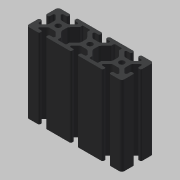
# Autodesk Inventor part: 40-4012-BLACK-FB
Saved by Autodesk Inventor 2013 SP2 (Build 170200200, 200)
## iProperties
Company: 80/20 Inc.
Created: 2014-04-23
Part Number: 40-4012-BLACK-FB
Material: Generic
Document SubType Name: Modeling
Designer: Ross Bowman
Density: 1 g/cm^3
Engineer: Ross Bowman
Catalog Web Link: 8020.net
Vendor: 80/20 Inc.
Mass: 225.385 g
Surface Area: 916.102 cm^2
Volume: 225.385 cm^3
Material: 6105-T5 Aluminum
Author: Ross Bowman
Keywords: 80/20 , 8020 , T-Slot , Extrusion
Autodesk Inventor part; units mm, degrees
ref_plane "YZ Plane" through (0, 0, 0) normal (1, 0, 0) x (0, 1, 0)
ref_plane "XZ Plane" through (0, 0, 0) normal (0, 1, 0) x (-1, 0, 0)
ref_plane "XY Plane" through (0, 0, 0) normal (0, 0, 1) x (1, 0, 0)
sketch "Sketch1" plane through (0, 0, 0) normal (0, 0, 1) x (1, 0, 0)
  circle A0 centre (40, 0) radius 3.4
  line L0 (9.0912, -6.0165) -> (14.2186, -11.1439)
  arc A1 (7.7, -2.6578) -> (9.0912, -6.0165) centre (12.45, -2.6578) ccw
  line L1 (7.7, 2.6265) -> (7.7, -2.6578)
  arc A2 (9.4012, 5.7139) -> (7.7, 2.6265) centre (12.4138, 2.0415) ccw
  line L2 (14.6946, 11.0074) -> (9.4012, 5.7139)
  arc A3 (14.6946, 11.0074) -> (15.0666, 11.9054) centre (13.7966, 11.9054) ccw
  line L3 (15.0666, 14.2735) -> (15.0666, 11.9054)
  arc A4 (16.3366, 15.68) -> (15.0666, 14.2735) centre (16.3292, 14.41) ccw
  line L4 (23.6634, 15.68) -> (16.3366, 15.68)
  arc A5 (24.9334, 14.41) -> (23.6634, 15.68) centre (23.6634, 14.41) ccw
  line L5 (24.9334, 12.0419) -> (24.9334, 14.41)
  arc A6 (24.9334, 12.0419) -> (25.3054, 11.1439) centre (26.2034, 12.0419) ccw
  line L6 (30.5988, 5.8505) -> (25.3054, 11.1439)
  arc A7 (32.3, 2.6265) -> (30.5988, 5.8505) centre (27.57, 2.1914) ccw
  line L7 (32.3, -2.6578) -> (32.3, 2.6265)
  arc A8 (30.9088, -6.0165) -> (32.3, -2.6578) centre (27.55, -2.6578) ccw
  line L8 (25.7814, -11.1439) -> (30.9088, -6.0165)
  arc A9 (25.7814, -11.1439) -> (25.4094, -12.0419) centre (26.6794, -12.0419) ccw
  line L9 (25.4094, -14.41) -> (25.4094, -12.0419)
  arc A10 (24.1394, -15.68) -> (25.4094, -14.41) centre (24.1394, -14.41) ccw
  line L10 (15.8606, -15.68) -> (24.1394, -15.68)
  arc A11 (14.5906, -14.41) -> (15.8606, -15.68) centre (15.8606, -14.41) ccw
  line L11 (14.5906, -12.0419) -> (14.5906, -14.41)
  arc A12 (14.5906, -12.0419) -> (14.2186, -11.1439) centre (13.3206, -12.0419) ccw
  circle A13 centre (0, 0) radius 3.4
  line L12 (-30.9088, -5.384) -> (-25.7814, -10.5113)
  arc A14 (-32.3, -2.0252) -> (-30.9088, -5.384) centre (-27.55, -2.0252) ccw
  line L13 (-32.3, 3.2591) -> (-32.3, -2.0252)
  arc A15 (-30.5988, 6.3465) -> (-32.3, 3.2591) centre (-27.5862, 2.6741) ccw
  line L14 (-25.3054, 11.6399) -> (-30.5988, 6.3465)
  arc A16 (-25.3054, 11.6399) -> (-24.9334, 12.538) centre (-26.2034, 12.538) ccw
  line L15 (-24.9334, 14.9061) -> (-24.9334, 12.538)
  arc A17 (-23.6634, 15.68) -> (-24.9334, 14.9061) centre (-23.7626, 14.4139) ccw
  line L16 (-16.3366, 15.68) -> (-23.6634, 15.68)
  arc A18 (-15.0666, 14.41) -> (-16.3366, 15.68) centre (-16.3366, 14.41) ccw
  line L17 (-15.0666, 12.0419) -> (-15.0666, 14.41)
  arc A19 (-15.0666, 12.0419) -> (-14.6946, 11.1439) centre (-13.7966, 12.0419) ccw
  line L18 (-9.4012, 5.8505) -> (-14.6946, 11.1439)
  arc A20 (-7.7, 2.6265) -> (-9.4012, 5.8505) centre (-12.43, 2.1914) ccw
  line L19 (-7.7, -2.6578) -> (-7.7, 2.6265)
  arc A21 (-9.0912, -6.0165) -> (-7.7, -2.6578) centre (-12.45, -2.6578) ccw
  line L20 (-14.2186, -11.1439) -> (-9.0912, -6.0165)
  arc A22 (-14.2186, -11.1439) -> (-14.5906, -12.0419) centre (-13.3206, -12.0419) ccw
  line L21 (-14.5906, -14.41) -> (-14.5906, -12.0419)
  arc A23 (-15.8606, -15.68) -> (-14.5906, -14.41) centre (-15.8606, -14.41) ccw
  line L22 (-24.1394, -15.68) -> (-15.8606, -15.68)
  arc A24 (-25.4094, -14.41) -> (-24.1394, -15.68) centre (-24.1394, -14.41) ccw
  line L23 (-25.4094, -11.4093) -> (-25.4094, -14.41)
  arc A25 (-25.4094, -11.4093) -> (-25.7814, -10.5113) centre (-26.6794, -11.4093) ccw
  circle A26 centre (-40, 0) radius 3.4
  arc A27 (-5.63, -20) -> (-4.06, -18.43) centre (-5.63, -18.43) ccw
  line L24 (-4.06, -18.43) -> (-4.06, -17.2093)
  arc A28 (-4.06, -17.2093) -> (-5.63, -15.68) centre (-5.6295, -17.25) ccw
  line L25 (-5.63, -15.68) -> (-8.7404, -15.68)
  arc A29 (-10.3104, -14.11) -> (-8.7404, -15.68) centre (-8.7404, -14.11) ccw
  line L26 (-10.3104, -14.11) -> (-10.3104, -13.7197)
  arc A30 (-10.0878, -13.1823) -> (-10.3104, -13.7197) centre (-9.5504, -13.7197) ccw
  line L27 (-10.0878, -13.1823) -> (-6.3105, -9.405)
  arc A31 (-3.3425, -7.7407) -> (-6.3105, -9.405) centre (-2.6575, -12.4411) ccw
  line L28 (-3.3425, -7.7407) -> (3.3406, -7.7407)
  arc A32 (6.3086, -9.405) -> (3.3406, -7.7407) centre (2.6556, -12.4411) ccw
  line L29 (6.3086, -9.405) -> (10.037, -13.1334)
  arc A33 (10.2596, -13.6708) -> (10.037, -13.1334) centre (9.4996, -13.6708) ccw
  line L30 (10.2596, -13.6708) -> (10.2596, -14.11)
  arc A34 (8.6896, -15.68) -> (10.2596, -14.11) centre (8.6896, -14.11) ccw
  line L31 (8.6896, -15.68) -> (5.5792, -15.68)
  arc A35 (5.5792, -15.68) -> (4.0092, -17.2093) centre (5.5787, -17.25) ccw
  line L32 (4.0092, -17.2093) -> (4.0092, -18.43)
  arc A36 (4.0092, -18.43) -> (5.5792, -20) centre (5.5792, -18.43) ccw
  line L33 (5.5792, -20) -> (34.3192, -20)
  arc A37 (34.3192, -20) -> (35.8892, -18.43) centre (34.3192, -18.43) ccw
  line L34 (35.8892, -18.43) -> (35.8892, -17.2093)
  arc A38 (35.8892, -17.2093) -> (34.3192, -15.68) centre (34.3197, -17.25) ccw
  line L35 (34.3192, -15.68) -> (31.2088, -15.68)
  arc A39 (29.6886, -14.0552) -> (31.2088, -15.68) centre (31.2577, -14.1108) ccw
  line L36 (29.6886, -14.0552) -> (29.6886, -13.6708)
  arc A40 (29.9112, -13.1334) -> (29.6886, -13.6708) centre (30.4486, -13.6708) ccw
  line L37 (29.9112, -13.1334) -> (33.6397, -9.405)
  arc A41 (36.6076, -7.7407) -> (33.6397, -9.405) centre (37.2927, -12.4411) ccw
  line L38 (36.6076, -7.7407) -> (43.2907, -7.7407)
  arc A42 (46.2587, -9.405) -> (43.2907, -7.7407) centre (42.6057, -12.4411) ccw
  line L39 (46.2587, -9.405) -> (50.036, -13.1823)
  arc A43 (50.2586, -13.7197) -> (50.036, -13.1823) centre (49.4986, -13.7197) ccw
  line L40 (50.2586, -13.7197) -> (50.2586, -14.0552)
  arc A44 (48.6896, -15.68) -> (50.2586, -14.0552) centre (48.6896, -14.11) ccw
  line L41 (48.6896, -15.68) -> (45.5792, -15.68)
  arc A45 (45.5792, -15.68) -> (44.0092, -17.2093) centre (45.5787, -17.25) ccw
  line L42 (44.0092, -17.2093) -> (44.0092, -18.4389)
  arc A46 (44.0092, -18.4389) -> (45.7462, -20) centre (45.5792, -18.4389) ccw
  line L43 (45.7462, -20) -> (57.0066, -20)
  arc A47 (57.0066, -20) -> (60, -16.83) centre (56.83, -16.8349) ccw
  line L44 (60, -16.83) -> (60, -5.5696)
  arc A48 (60, -5.5696) -> (58.43, -3.9996) centre (58.43, -5.5696) ccw
  line L45 (58.43, -3.9996) -> (57.25, -3.9996)
  arc A49 (57.25, -3.9996) -> (55.68, -5.5696) centre (57.25, -5.5696) ccw
  line L46 (55.68, -5.5696) -> (55.68, -8.4722)
  arc A50 (54.111, -10.097) -> (55.68, -8.4722) centre (54.111, -8.527) ccw
  line L47 (54.111, -10.097) -> (53.4665, -10.097)
  arc A51 (52.9291, -9.8744) -> (53.4665, -10.097) centre (53.4665, -9.337) ccw
  line L48 (52.9291, -9.8744) -> (48.9155, -5.8608)
  arc A52 (47.7, -2.502) -> (48.9155, -5.8608) centre (52.4465, -2.6836) ccw
  line L49 (47.7, -2.502) -> (47.7, 2.571)
  arc A53 (49.0111, 5.9564) -> (47.7, 2.571) centre (52.4488, 2.6785) ccw
  line L50 (49.0111, 5.9564) -> (53.1886, 10.1339)
  arc A54 (53.726, 10.3565) -> (53.1886, 10.1339) centre (53.726, 9.5965) ccw
  line L51 (53.726, 10.3565) -> (54.11, 10.3565)
  arc A55 (55.68, 8.7865) -> (54.11, 10.3565) centre (54.11, 8.7865) ccw
  line L52 (55.68, 8.7865) -> (55.68, 5.8839)
  arc A56 (55.68, 5.8839) -> (57.1443, 4.1259) centre (57.2384, 5.693) ccw
  line L53 (57.1443, 4.1259) -> (58.3243, 4.1259)
  arc A57 (58.3243, 4.1259) -> (60, 5.5825) centre (58.4338, 5.692) ccw
  line L54 (60, 5.5825) -> (60, 16.8406)
  arc A58 (60, 16.8406) -> (56.83, 20) centre (56.83, 16.83) ccw
  line L55 (56.83, 20) -> (45.5696, 20)
  arc A59 (45.5696, 20) -> (43.9996, 18.43) centre (45.5696, 18.43) ccw
  line L56 (43.9996, 18.43) -> (43.9996, 17.25)
  arc A60 (43.9996, 17.25) -> (45.5696, 15.68) centre (45.5696, 17.25) ccw
  line L57 (45.5696, 15.68) -> (48.715, 15.68)
  arc A61 (50.285, 14.11) -> (48.715, 15.68) centre (48.715, 14.11) ccw
  line L58 (50.285, 14.11) -> (50.285, 13.6545)
  arc A62 (50.0624, 13.1171) -> (50.285, 13.6545) centre (49.525, 13.6545) ccw
  line L59 (50.0624, 13.1171) -> (45.9081, 8.9628)
  arc A63 (42.5494, 7.7) -> (45.9081, 8.9628) centre (42.6809, 12.4482) ccw
  line L60 (42.5494, 7.7) -> (37.4506, 7.7)
  arc A64 (34.0919, 8.9628) -> (37.4506, 7.7) centre (37.3191, 12.4482) ccw
  line L61 (34.0919, 8.9628) -> (29.9376, 13.1171)
  arc A65 (29.715, 13.6545) -> (29.9376, 13.1171) centre (30.475, 13.6545) ccw
  line L62 (29.715, 13.6545) -> (29.715, 14.11)
  arc A66 (31.285, 15.68) -> (29.715, 14.11) centre (31.285, 14.11) ccw
  line L63 (31.285, 15.68) -> (34.5165, 15.68)
  arc A67 (34.5165, 15.68) -> (36.0865, 17.25) centre (34.5165, 17.25) ccw
  line L64 (36.0865, 17.25) -> (36.0865, 18.43)
  arc A68 (36.0865, 18.43) -> (34.5165, 20) centre (34.5165, 18.43) ccw
  line L65 (34.5165, 20) -> (5.4816, 20)
  arc A69 (5.4816, 20) -> (3.9116, 18.43) centre (5.4816, 18.43) ccw
  line L66 (3.9116, 18.43) -> (3.9116, 17.25)
  arc A70 (3.9116, 17.25) -> (5.4816, 15.68) centre (5.4816, 17.25) ccw
  line L67 (5.4816, 15.68) -> (8.715, 15.68)
  arc A71 (10.285, 14.11) -> (8.715, 15.68) centre (8.715, 14.11) ccw
  line L68 (10.285, 14.11) -> (10.285, 13.6545)
  arc A72 (10.0624, 13.1171) -> (10.285, 13.6545) centre (9.525, 13.6545) ccw
  line L69 (10.0624, 13.1171) -> (5.9081, 8.9628)
  arc A73 (2.5494, 7.7) -> (5.9081, 8.9628) centre (2.6809, 12.4482) ccw
  line L70 (2.5494, 7.7) -> (-2.5494, 7.7)
  arc A74 (-5.9081, 8.9628) -> (-2.5494, 7.7) centre (-2.6809, 12.4482) ccw
  line L71 (-5.9081, 8.9628) -> (-10.0624, 13.1171)
  arc A75 (-10.285, 13.6545) -> (-10.0624, 13.1171) centre (-9.525, 13.6545) ccw
  line L72 (-10.285, 13.6545) -> (-10.285, 14.11)
  arc A76 (-8.715, 15.68) -> (-10.285, 14.11) centre (-8.715, 14.11) ccw
  line L73 (-8.715, 15.68) -> (-5.4835, 15.68)
  arc A77 (-5.4835, 15.68) -> (-3.9135, 17.25) centre (-5.4835, 17.25) ccw
  line L74 (-3.9135, 17.25) -> (-3.9135, 18.43)
  arc A78 (-3.9135, 18.43) -> (-5.4835, 20) centre (-5.4835, 18.43) ccw
  line L75 (-5.4835, 20) -> (-34.5165, 20)
  line L76 (-36.0865, 18.43) -> (-36.0865, 17.2476)
  arc A79 (-36.0865, 17.2476) -> (-34.5165, 15.68) centre (-34.5165, 17.25) ccw
  line L77 (-34.5165, 15.68) -> (-31.285, 15.68)
  arc A80 (-29.715, 14.11) -> (-31.285, 15.68) centre (-31.285, 14.11) ccw
  line L78 (-29.715, 14.11) -> (-29.715, 13.6545)
  arc A81 (-29.9376, 13.1171) -> (-29.715, 13.6545) centre (-30.475, 13.6545) ccw
  line L79 (-29.9376, 13.1171) -> (-34.0919, 8.9628)
  arc A82 (-37.4506, 7.7) -> (-34.0919, 8.9628) centre (-37.3191, 12.4482) ccw
  line L80 (-37.4506, 7.7) -> (-42.5494, 7.7)
  arc A83 (-45.9081, 8.9628) -> (-42.5494, 7.7) centre (-42.6809, 12.4482) ccw
  line L81 (-45.9081, 8.9628) -> (-50.0624, 13.1171)
  arc A84 (-50.285, 13.6545) -> (-50.0624, 13.1171) centre (-49.525, 13.6545) ccw
  line L82 (-50.285, 13.6545) -> (-50.285, 14.11)
  arc A85 (-48.715, 15.68) -> (-50.285, 14.11) centre (-48.715, 14.11) ccw
  line L83 (-48.715, 15.68) -> (-45.5696, 15.68)
  arc A86 (-45.5696, 15.68) -> (-43.9996, 17.25) centre (-45.5696, 17.25) ccw
  line L84 (-43.9996, 17.25) -> (-43.9996, 18.43)
  arc A87 (-43.9996, 18.43) -> (-45.5696, 20) centre (-45.5696, 18.43) ccw
  line L85 (-45.5696, 20) -> (-56.83, 20)
  arc A88 (-56.83, 20) -> (-60, 16.8406) centre (-56.83, 16.83) ccw
  line L86 (-60, 16.8406) -> (-60, 5.5825)
  arc A89 (-60, 5.5825) -> (-58.3243, 4.1259) centre (-58.4338, 5.692) ccw
  line L87 (-58.3243, 4.1259) -> (-57.1443, 4.1259)
  arc A90 (-57.1443, 4.1259) -> (-55.68, 5.8839) centre (-57.2384, 5.693) ccw
  line L88 (-55.68, 5.8839) -> (-55.68, 8.7865)
  arc A91 (-54.11, 10.3565) -> (-55.68, 8.7865) centre (-54.11, 8.7865) ccw
  line L89 (-54.11, 10.3565) -> (-53.726, 10.3565)
  arc A92 (-53.1886, 10.1339) -> (-53.726, 10.3565) centre (-53.726, 9.5965) ccw
  line L90 (-53.1886, 10.1339) -> (-49.0111, 5.9564)
  arc A93 (-47.7, 2.571) -> (-49.0111, 5.9564) centre (-52.4488, 2.6785) ccw
  line L91 (-47.7, 2.571) -> (-47.7, -2.502)
  arc A94 (-48.9155, -5.8608) -> (-47.7, -2.502) centre (-52.4465, -2.6836) ccw
  line L92 (-48.9155, -5.8608) -> (-52.9291, -9.8744)
  arc A95 (-53.4665, -10.097) -> (-52.9291, -9.8744) centre (-53.4665, -9.337) ccw
  line L93 (-53.4665, -10.097) -> (-54.111, -10.097)
  arc A96 (-55.68, -8.4722) -> (-54.111, -10.097) centre (-54.111, -8.527) ccw
  line L94 (-55.68, -8.4722) -> (-55.68, -5.5696)
  arc A97 (-55.68, -5.5696) -> (-57.25, -3.9996) centre (-57.25, -5.5696) ccw
  line L95 (-57.25, -3.9996) -> (-58.43, -3.9996)
  arc A98 (-58.43, -3.9996) -> (-60, -5.5696) centre (-58.43, -5.5696) ccw
  line L96 (-60, -5.5696) -> (-60, -16.83)
  arc A99 (-60, -16.83) -> (-57.0574, -20) centre (-56.83, -16.8382) ccw
  line L97 (-57.0574, -20) -> (-45.797, -20)
  arc A100 (-45.797, -20) -> (-44.06, -18.4389) centre (-45.63, -18.4389) ccw
  line L98 (-44.06, -18.4389) -> (-44.06, -17.25)
  arc A101 (-44.06, -17.25) -> (-45.63, -15.68) centre (-45.63, -17.25) ccw
  line L99 (-45.63, -15.68) -> (-48.7404, -15.68)
  arc A102 (-50.3104, -14.11) -> (-48.7404, -15.68) centre (-48.7404, -14.11) ccw
  line L100 (-50.3104, -14.11) -> (-50.3104, -13.7197)
  arc A103 (-50.0878, -13.1823) -> (-50.3104, -13.7197) centre (-49.5504, -13.7197) ccw
  line L101 (-50.0878, -13.1823) -> (-46.3105, -9.405)
  arc A104 (-43.3425, -7.7407) -> (-46.3105, -9.405) centre (-42.6575, -12.4411) ccw
  line L102 (-43.3425, -7.7407) -> (-36.6594, -7.7407)
  arc A105 (-33.6914, -9.405) -> (-36.6594, -7.7407) centre (-37.3444, -12.4411) ccw
  line L103 (-33.6914, -9.405) -> (-29.9611, -13.1353)
  arc A106 (-29.7385, -13.6727) -> (-29.9611, -13.1353) centre (-30.4985, -13.6727) ccw
  line L104 (-29.7385, -13.6727) -> (-29.7385, -14.1108)
  arc A107 (-31.2596, -15.68) -> (-29.7385, -14.1108) centre (-31.3085, -14.1108) ccw
  line L105 (-31.2596, -15.68) -> (-34.37, -15.68)
  arc A108 (-34.37, -15.68) -> (-35.94, -17.25) centre (-34.37, -17.25) ccw
  line L106 (-35.94, -17.25) -> (-35.94, -18.43)
  arc A109 (-35.94, -18.43) -> (-34.37, -20) centre (-34.37, -18.43) ccw
  line L107 (-34.37, -20) -> (-5.63, -20)
  arc A110 (-34.5165, 20) -> (-36.0865, 18.43) centre (-34.5165, 18.43) ccw
  constraints: 216 end point, 216 point on circle, 111 centre point
extrude "Extrusion1" add sketch "Sketch1" against normal blind 100
body "Solid1"
